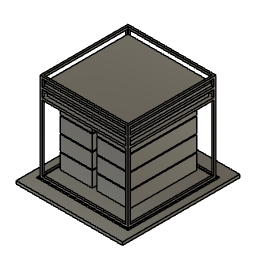
_2Boards_ED.5db593b0-eb79-4f9a-a5e3-c8a486b85028 (Autodesk Fusion 360 design; units mm, degrees)
Autodesk Fusion 360 part; units mm, degrees
note: some values were not read from the file. Chosen so that the rebuilt part matches the saved one: which bodies a step acts on. Set by a fixed rule: which sketch regions a step uses.
sketch "Sketch1" plane through (0, 0, 0) normal (0, 0, 1) x (1, 0, 0)
  line L0 (29, 32) -> (-29, 32)
  line L1 (-29, 32) -> (-29, -32)
  line L2 (-29, -32) -> (29, -32)
  line L3 (29, -32) -> (29, 32)
  line L4 (29, 32) -> (-29, -32) construction
  line L5 (-29, 32) -> (29, -32) construction
  dimension "d1" = 64
  dimension "d2" = 58
  constraint perpendicular L0 L1
  constraint parallel L0 L2
  constraint parallel L1 L3
  constraint horizontal L0
  constraint coincident L4 origin
  constraint coincident L5 origin
  measures "d1" distance of L0.end L1.end
  measures "d2" distance of L1.end L2.end
extrude "Extrude1" add sketch "Sketch1" along normal blind 1.6 makes body 1
sketch "Sketch2" plane through (0, 0, 1.6) normal (0, 0, 1) x (-1, 0, 0)
  line L0 (-29, 32) -> (-29, -32)
  line L1 (-29, -32) -> (29, -32)
  line L2 (29, -32) -> (29, 32)
  line L3 (29, 32) -> (-29, 32)
  line L4 (-25, -25) -> (25, -25)
  line L5 (25, -25) -> (25, 25)
  line L6 (25, 25) -> (-25, 25)
  line L7 (-25, 25) -> (-25, -25)
  line L8 (-25, -25) -> (25, 25) construction
  line L9 (25, -25) -> (-25, 25) construction
  line L10 (-24.2, -24.2) -> (24.2, -24.2)
  line L11 (24.2, -24.2) -> (24.2, 24.2)
  line L12 (24.2, 24.2) -> (-24.2, 24.2)
  line L13 (-24.2, 24.2) -> (-24.2, -24.2)
  line L14 (-24.2, -24.2) -> (24.2, 24.2) construction
  line L15 (24.2, -24.2) -> (-24.2, 24.2) construction
  dimension "d5" = 50
  dimension "d6" = 50
  dimension "d7" = 48.4
  dimension "d8" = 48.4
  constraint perpendicular L4 L5
  constraint parallel L4 L6
  constraint parallel L5 L7
  constraint horizontal L4
  constraint coincident L8 origin
  constraint coincident L9 origin
  constraint perpendicular L10 L11
  constraint parallel L10 L12
  constraint parallel L11 L13
  constraint horizontal L10
  constraint coincident L14 origin
  constraint coincident L15 origin
  measures "d5" distance of L4.start L4.end
  measures "d6" distance of L4.start L6.end
  measures "d7" distance of L10.start L12.end
  measures "d8" distance of L11.end L12.end
extrude "Extrude2" cut sketch "Sketch2" against normal blind 0.8 contours L4 L5 L6 L7 bodies 1
sketch "Sketch3" plane through (0, 0, 1.6) normal (0, 0, 1) x (-1, 0, 0)
  line L0 (24.2, 24.2) -> (-24.2, 24.2)
  line L1 (-24.2, 24.2) -> (-24.2, -24.2)
  line L2 (-24.2, -24.2) -> (24.2, -24.2)
  line L3 (24.2, -24.2) -> (24.2, 24.2)
  line L4 (-23, -23) -> (23, -23)
  line L5 (23, -23) -> (23, 23)
  line L6 (23, 23) -> (-23, 23)
  line L7 (-23, 23) -> (-23, -23)
  line L8 (-23, -23) -> (23, 23) construction
  line L9 (23, -23) -> (-23, 23) construction
  dimension "d11" = 46
  dimension "d12" = 46
  constraint perpendicular L4 L5
  constraint parallel L4 L6
  constraint parallel L5 L7
  constraint horizontal L4
  constraint coincident L8 origin
  constraint coincident L9 origin
  measures "d11" distance of L4.start L4.end
  measures "d12" distance of L4.start L6.end
extrude "Extrude3" cut sketch "Sketch3" against normal blind 1.6 contours L4 L5 L6 L7 bodies 1
sketch "Sketch4" plane through (0, 0, 0) normal (0, 0, 1) x (1, 0, 0)
  line L0 (23, 23) -> (-23, -23) construction
  line L1 (-23, 23) -> (23, -23) construction
  line L2 (18, 23) -> (23, 18)
  line L3 (18, -23) -> (23, -18)
  line L4 (-23, -18) -> (-18, -23)
  line L5 (-23, 23) -> (-23, 18)
  line L6 (-23, -18) -> (-23, -23)
  line L7 (23, 23) -> (18, 23)
  line L8 (-18, 23) -> (-23, 23)
  line L9 (23, -23) -> (23, -18)
  line L10 (23, 18) -> (23, 23)
  line L11 (-23, -23) -> (-18, -23)
  line L12 (18, -23) -> (23, -23)
  line L13 (-23, 18) -> (-18, 23)
  constraint perpendicular L5 L7
  constraint parallel L7 L11
  constraint parallel L5 L9
  constraint horizontal L7
  constraint coincident L0 origin
  constraint coincident L1 origin
  constraint coincident L2.end L9
  constraint perpendicular L0 L2
  constraint coincident L3.start L11
  constraint perpendicular L1 L3
  constraint coincident L4.start L5
  constraint perpendicular L0 L4
  constraint collinear L5 L6
  constraint collinear L7 L8
  constraint collinear L9 L10
  constraint collinear L11 L12
  constraint perpendicular L1 L13
extrude "Extrude4" add sketch "Sketch4" along normal blind 0.8 bodies 1
sketch "Sketch6" plane through (0, 0, 0.8) normal (0, 0, 1) x (-1, 0, 0)
  line L0 (18, -23) -> (23, -23)
  line L1 (23, -23) -> (23, -18)
  line L2 (-23, -23) -> (23, -23)
  line L3 (23, -23) -> (23, 23)
  line L4 (23, 23) -> (-23, 23)
  line L5 (-23, 23) -> (-23, -23)
  line L6 (-23, -23) -> (23, 23) construction
  line L7 (23, -23) -> (-23, 23) construction
  constraint perpendicular L2 L3
  constraint parallel L2 L4
  constraint parallel L3 L5
  constraint horizontal L2
  constraint coincident L6 origin
  constraint coincident L7 origin
extrude "Extrude5" add sketch "Sketch6" along normal blind 1.6 separate body makes body 2
sketch "Sketch7" plane through (0, 0, 0) normal (0, 0, 1) x (1, 0, 0)
  line L0 (24, 24) -> (-24, 24)
  line L1 (-24, 24) -> (-24, -24)
  line L2 (-24, -24) -> (24, -24)
  line L3 (24, -24) -> (24, 24)
  line L4 (24, 24) -> (-24, -24) construction
  line L5 (-24, 24) -> (24, -24) construction
  line L6 (23, 23) -> (-23, 23)
  line L7 (-23, 23) -> (-23, -23)
  line L8 (-23, -23) -> (23, -23)
  line L9 (23, -23) -> (23, 23)
  line L10 (23, 23) -> (-23, -23) construction
  line L11 (-23, 23) -> (23, -23) construction
  constraint perpendicular L0 L1
  constraint parallel L0 L2
  constraint parallel L1 L3
  constraint horizontal L0
  constraint coincident L4 origin
  constraint coincident L5 origin
  constraint perpendicular L6 L7
  constraint parallel L6 L8
  constraint parallel L7 L9
  constraint horizontal L6
  constraint coincident L4 L6.start
  constraint coincident L10 origin
  constraint coincident L11 origin
extrude "Extrude6" add sketch "Sketch7" along normal blind 48.4 from surface at 1.6 separate body makes body 3
sketch "Sketch8" plane through (0, -24, 0) normal (0, -1, 0) x (1, 0, 0)
  line L0 (-24, 1.6) -> (24, 1.6)
  line L1 (24, 1.6) -> (24, 50)
  line L2 (24, 50) -> (-24, 50)
  line L3 (-24, 50) -> (-24, 1.6)
  line L4 (-22.8, 2.8) -> (22.8, 2.8)
  line L5 (22.8, 2.8) -> (22.8, 48.8)
  line L6 (22.8, 48.8) -> (-22.8, 48.8)
  line L7 (-22.8, 48.8) -> (-22.8, 2.8)
  line L8 (-22.8, 45) -> (22.8, 45)
  line L9 (-22.8, 43.8) -> (22.8, 43.8)
  line L10 (-22.8, 40) -> (22.8, 40)
  line L11 (-22.8, 38.8) -> (22.8, 38.8)
  dimension "d27" = 1.2
  dimension "d28" = 1.2
  dimension "d29" = 1.2
  dimension "d30" = 1.2
  dimension "d31" = 3.8
  dimension "d32" = 1.2
  dimension "d33" = 3.8
  dimension "d34" = 1.2
  constraint coincident L7 L8.start
  constraint coincident L5 L8.end
  constraint perpendicular L5 L8
  constraint coincident L7 L9.start
  constraint coincident L5 L9.end
  constraint perpendicular L5 L9
  constraint coincident L7 L10.start
  constraint coincident L5 L10.end
  constraint perpendicular L5 L10
  constraint coincident L7 L11.start
  constraint coincident L5 L11.end
  constraint perpendicular L5 L11
  measures "d27" distance of L2 L6
  measures "d28" distance of L3 L7
  measures "d29" distance of L1 L5
  measures "d30" distance of L0 L4
  measures "d31" distance of L6 L8
  measures "d32" distance of L8 L9
  measures "d33" distance of L9 L10
  measures "d34" distance of L10 L11
extrude "Extrude7" cut sketch "Sketch8" against normal blind 1.2 contours L4 L5 L7 L11 | L5 L7 L10 L11 | L5 L7 L9 L10 | L5 L7 L8 L9 | L5 L6 L7 L8 bodies 3
pattern_circular "C-Pattern1" count 4 over 360 about axis through (0, 0, 1.75) along (0, 0, 1) of "Extrude7"
extrude "Extrude8" add sketch "Sketch8" against normal blind 1.2 contours L5 L7 L10 L11 | L5 L7 L8 L9 bodies 3
pattern_circular "C-Pattern2" count 4 over 360 about axis through (0, 0, 1.75) along (0, 0, 1) of "Extrude8"
extrude "Extrude9" cut sketch "Sketch8" against normal blind 2 contours L5 L7 L10 L11 | L5 L7 L8 L9 bodies 3
extrude "Extrude10" add sketch "Sketch8" against normal blind 2 contours L5 L7 L10 L11 | L5 L7 L8 L9 bodies 3
pattern_circular "C-Pattern3" count 4 over 360 about axis through (0, 0, 1.75) along (0, 0, 1) of "Extrude10"
sketch "Sketch9" plane through (0, 0, 45) normal (0, 0, 1) x (-1, 0, 0)
  line L0 (22.8, 22.8) -> (22.8, 23)
  line L1 (22.8, 23) -> (22.8, 24)
  line L2 (22.8, 24) -> (-22.8, 24)
  line L3 (-22.8, 24) -> (-22.8, 23)
  line L4 (-22.8, 23) -> (-22.8, 22.8)
  line L5 (-22.8, 22.8) -> (-23, 22.8)
  line L6 (-23, 22.8) -> (-24, 22.8)
  line L7 (-24, 22.8) -> (-24, -22.8)
  line L8 (-24, -22.8) -> (-23, -22.8)
  line L9 (-23, -22.8) -> (-22.8, -22.8)
  line L10 (-22.8, -22.8) -> (-22.8, -23)
  line L11 (-22.8, -23) -> (-22.8, -24)
  line L12 (-22.8, -24) -> (22.8, -24)
  line L13 (22.8, -24) -> (22.8, -23)
  line L14 (22.8, -23) -> (22.8, -22.8)
  line L15 (22.8, -22.8) -> (23, -22.8)
  line L16 (23, -22.8) -> (24, -22.8)
  line L17 (24, -22.8) -> (24, 22.8)
  line L18 (24, 22.8) -> (23, 22.8)
  line L19 (23, 22.8) -> (22.8, 22.8)
  line L20 (-23, 23) -> (23, 23)
  line L21 (23, 23) -> (23, -23)
  line L22 (23, -23) -> (-23, -23)
  line L23 (-23, -23) -> (-23, 23)
  line L24 (-23, 23) -> (23, -23) construction
  line L25 (23, 23) -> (-23, -23) construction
  line L26 (-22.8, -22.8) -> (22.8, -22.8)
  line L27 (22.8, -22.8) -> (22.8, 22.8)
  line L28 (22.8, 22.8) -> (-22.8, 22.8)
  line L29 (-22.8, 22.8) -> (-22.8, -22.8)
  line L30 (-22.8, -22.8) -> (22.8, 22.8) construction
  line L31 (22.8, -22.8) -> (-22.8, 22.8) construction
  constraint perpendicular L20 L21
  constraint parallel L20 L22
  constraint parallel L21 L23
  constraint horizontal L20
  constraint coincident L24 origin
  constraint coincident L25 origin
  constraint perpendicular L26 L27
  constraint parallel L26 L28
  constraint parallel L27 L29
  constraint horizontal L26
  constraint coincident L9.end L10.start
  constraint coincident L30 origin
  constraint coincident L31 origin
extrude "Extrude13" add sketch "Sketch9" along normal blind 1.6 separate body contours L26 L27 L28 L29 makes body 4
sketch "Sketch10" plane through (0, 0, 40) normal (0, 0, 1) x (-1, 0, 0)
  line L0 (22.8, 22.8) -> (22.8, 23)
  line L1 (22.8, 23) -> (22.8, 24)
  line L2 (22.8, 24) -> (-22.8, 24)
  line L3 (-22.8, 24) -> (-22.8, 23)
  line L4 (-22.8, 23) -> (-22.8, 22.8)
  line L5 (-22.8, 22.8) -> (-23, 22.8)
  line L6 (-23, 22.8) -> (-24, 22.8)
  line L7 (-24, 22.8) -> (-24, -22.8)
  line L8 (-24, -22.8) -> (-23, -22.8)
  line L9 (-23, -22.8) -> (-22.8, -22.8)
  line L10 (-22.8, -22.8) -> (-22.8, -23)
  line L11 (-22.8, -23) -> (-22.8, -24)
  line L12 (-22.8, -24) -> (22.8, -24)
  line L13 (22.8, -24) -> (22.8, -23)
  line L14 (22.8, -23) -> (22.8, -22.8)
  line L15 (22.8, -22.8) -> (23, -22.8)
  line L16 (23, -22.8) -> (24, -22.8)
  line L17 (24, -22.8) -> (24, 22.8)
  line L18 (24, 22.8) -> (23, 22.8)
  line L19 (23, 22.8) -> (22.8, 22.8)
  line L20 (22, 22) -> (22, -22)
  line L21 (22, -22) -> (-22, -22)
  line L22 (-22, -22) -> (-22, 22)
  line L23 (-22, 22) -> (22, 22)
  line L24 (-23, -22.8) -> (23, -22.8)
  line L25 (23, -22.8) -> (23, 22.8)
  line L26 (23, 22.8) -> (-23, 22.8)
  line L27 (-23, 22.8) -> (-23, -22.8)
  line L28 (-23, -22.8) -> (23, 22.8) construction
  line L29 (23, -22.8) -> (-23, 22.8) construction
  constraint perpendicular L24 L25
  constraint parallel L24 L26
  constraint parallel L25 L27
  constraint horizontal L24
  constraint coincident L8.end L9.start
  constraint coincident L28 origin
  constraint coincident L29 origin
extrude "Extrude14" add sketch "Sketch10" along normal blind 1.6 separate body contours L20 L21 L22 L23 makes body 5
sketch "Sketch11" plane through (0, 0, 0) normal (0, 0, 1) x (1, 0, 0)
  line L0 (-20.8, 20.8) -> (-3.3, 20.8)
  line L1 (-3.3, 20.8) -> (-3.3, -16.2)
  line L2 (-3.3, -16.2) -> (-20.8, -16.2)
  line L3 (-20.8, -16.2) -> (-20.8, 20.8)
  line L4 (22.8, 22.8) -> (-22.8, 22.8)
  line L5 (-22.8, 22.8) -> (-22.8, -22.8)
  dimension "d53" = 17.5
  dimension "d54" = 37
  dimension "d55" = 2
  dimension "d56" = 2
  constraint horizontal L0
  constraint vertical L1
  constraint horizontal L2
  constraint vertical L3
  measures "d53" distance of L0.start L0.end
  measures "d54" distance of L0.start L2.end
  measures "d55" distance of L0 L4
  measures "d56" distance of L3 L5
extrude "Extrude15" add sketch "Sketch11" along normal blind 8.2 from surface at 3 separate body makes body 6
pattern_linear "R-Pattern1" count 3 spacing 12 along (0, 0, 1) of bodies 6 makes body 7 at (-14.9667, -3.8667, 15) makes body 8 at (-14.9667, -3.8667, 27)
pattern_linear "R-Pattern2" count 2 spacing 20 along (1, 0, 0) of bodies 6 7 8 makes body 9 at (5.0333, -3.8667, 27) makes body 10 at (5.0333, -3.8667, 3) makes body 11 at (5.0333, -3.8667, 15)
pattern_linear "R-Pattern3" count 4 spacing 8.6667 along (0, 0, 1) of bodies 6 makes body 12 at (-14.9667, -3.8667, 11.6667) makes body 13 at (-14.9667, -3.8667, 20.3333) makes body 14 at (-14.9667, -3.8667, 29)
pattern_linear "R-Pattern4" count 2 spacing 20 along (1, 0, 0) of bodies 6 14 12 13 makes body 15 at (5.0333, -3.8667, 20.3333) makes body 16 at (5.0333, -3.8667, 3) makes body 17 at (5.0333, -3.8667, 29) makes body 18 at (5.0333, -3.8667, 11.6667)
sketch "Sketch12" plane through (0, 0, 2.4) normal (0, 0, 1) x (-1, 0, 0)
  line L0 (-23, 23) -> (-23, -23)
  line L1 (-23, -23) -> (23, -23)
  line L2 (23, -23) -> (23, 23)
  line L3 (23, 23) -> (-23, 23)
  line L4 (21.6, -21.6) -> (-12.4, -21.6)
  line L5 (-12.4, -21.6) -> (-12.4, 21.7)
  line L6 (-12.4, 21.7) -> (21.6, 21.7)
  line L7 (21.6, 21.7) -> (21.6, -21.6)
  line L8 (-22.8, -22.8) -> (22.8, -22.8)
  line L9 (22.8, -22.8) -> (22.8, 22.8)
  dimension "d76" = 34
  dimension "d77" = 43.3
  dimension "d78" = 1.2
  dimension "d79" = 1.2
  constraint horizontal L4
  constraint vertical L5
  constraint horizontal L6
  constraint vertical L7
  measures "d76" distance of L4.start L4.end
  measures "d77" distance of L4.end L5.end
  measures "d78" distance of L4 L8
  measures "d79" distance of L7 L9
extrude "Extrude16" add sketch "Sketch12" along normal blind 6 separate body contours L4 L5 L6 L7 makes body 19
pattern_linear "R-Pattern5" count 5 spacing 6.25 along (0, 0, 1) of bodies 19 makes body 20 at (-10.2667, 7.1667, 8.65) makes body 21 at (-10.2667, 7.1667, 14.9) makes body 22 at (-10.2667, 7.1667, 21.15) makes body 23 at (-10.2667, 7.1667, 27.4)
equation "d7 = 50 mm - 1.6 mm"
equation "d8 = 50 mm - 1.6 mm"
equation "d20 = 50 mm - 1.6 mm"
equation "d31 = 5 mm - 1.2 mm"
equation "d33 = 5 mm - 1.2 mm"
named bodies: "Backplate", "Bottom board", "Scaffold", "Inner Board 2", "Inner Board 1", "AdaFruit", "AdaFruit (1)", "AdaFruit (2)", "AdaFruit (3)", "AdaFruit (2) (1)", "AdaFruit (4)", "AdaFruit (3) (1)", "AdaFruit (1) (1)", "SparkFun", "SparkFun (1) (1)", "SparkFun (1)", "SparkFun (3)", "SparkFun (4)"
